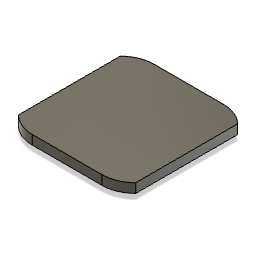
TopPanelWave v5 (Autodesk Fusion 360 design; units mm, degrees)
Autodesk Fusion 360 part; units mm, degrees
sketch "Sketch1" plane through (0, 0, 0) normal (0, 1, 0) x (1, 0, 0)
  line L0 (86, 73.5) -> (-86, 73.5)
  line L1 (-86, 73.5) -> (-86, -73.5)
  line L2 (-86, -73.5) -> (86, -73.5)
  line L3 (86, -73.5) -> (86, 73.5)
  line L4 (86, 73.5) -> (-86, -73.5) construction
  line L5 (-86, 73.5) -> (86, -73.5) construction
  line L6 (-77, -64.5) -> (77, -64.5)
  line L7 (77, -64.5) -> (77, 64.5)
  line L8 (77, 64.5) -> (-77, 64.5)
  line L9 (-77, 64.5) -> (-77, -64.5)
  line L10 (102, -89.5) -> (102, 89.5)
  line L11 (102, 89.5) -> (-102, 89.5)
  line L12 (-102, 89.5) -> (-102, -89.5)
  line L13 (-102, -89.5) -> (102, -89.5)
  dimension "d1" = 172
  dimension "d6" = 147
  dimension "d15" = 16
  constraint horizontal L0
  constraint perpendicular L0 L1
  constraint parallel L0 L2
  constraint parallel L1 L3
  constraint coincident L4 origin
  constraint coincident L5 origin
  measures "d1" distance of L1.end L2.end
  measures "d6" distance of L0.end L1.end
extrude "Extrude1" add sketch "Sketch1" along normal blind 9 contours L0 L1 L2 L3
ref_plane "WorkPlane1" through (0, 9, 0) normal (0, 1, 0) x (0, 0, 1)
sketch "Sketch2" plane through (0, 9, 0) normal (0, 1, 0) x (1, 0, 0)
  line L0 (-77, -64.5) -> (-77, 64.5)
  line L1 (-77, 64.5) -> (77, 64.5)
  line L2 (77, 64.5) -> (77, -64.5)
  line L3 (77, -64.5) -> (-77, -64.5)
  line L4 (86, -73.5) -> (86, 73.5)
  line L5 (86, 73.5) -> (-86, 73.5)
  line L6 (-86, 73.5) -> (-86, -73.5)
  line L7 (-86, -73.5) -> (86, -73.5)
  line L8 (95, -82.5) -> (95, 82.5)
  line L9 (95, 82.5) -> (-95, 82.5)
  line L10 (-95, 82.5) -> (-95, -82.5)
  line L11 (-95, -82.5) -> (95, -82.5)
  line L12 (-111, -98.5) -> (111, -98.5)
  line L13 (111, -98.5) -> (111, 98.5)
  line L14 (111, 98.5) -> (-111, 98.5)
  line L15 (-111, 98.5) -> (-111, -98.5)
  arc A0 (-56.3726, 98.5) -> (-111, 43.8726) centre (-56.3726, 43.8726) ccw
  arc A1 (-111, -43.8726) -> (-56.3726, -98.5) centre (-56.3726, -43.8726) ccw
  arc A2 (56.3726, -98.5) -> (111, -43.8726) centre (56.3726, -43.8726) ccw
  arc A3 (111, 43.8726) -> (56.3726, 98.5) centre (56.3726, 43.8726) ccw
  dimension "d11" = 9
  dimension "d16" = 25
  constraint coincident L9.end A0
  constraint coincident L14 A0.start
  constraint coincident L15 A0.end
  constraint coincident L10.end A1
  constraint coincident L12 A1.end
  constraint coincident L15 A1.start
  constraint coincident L8.start A2
  constraint coincident L13 A2.end
  constraint coincident L12 A2.start
  constraint coincident L8.end A3
  constraint coincident L13 A3.start
  constraint coincident L14 A3.end
  constraint tangent L14 A0
  constraint tangent L15 A0
  constraint tangent L15 A1
  constraint tangent L12 A1
  constraint tangent L12 A2
  constraint tangent L13 A2
  constraint tangent L13 A3
  constraint tangent L14 A3
extrude "Extrude2" add sketch "Sketch2" along normal blind 15 contours L0 L1 L2 L3 | L4 L5 L6 L7 | L8 L9 L10 L11 | L11 L12 A1 A2 | L9 L14 A0 A3
equation "d1 = CaseLength - 2 * SideWidth"
equation "CaseLength = 190 mm"
equation "CaseWidth = 165 mm"
equation "SideWidth = 9 mm"
equation "PanelHeight = 15 mm"
equation "d6 = CaseWidth - 2 * SideWidth"
equation "d7 = -SideWidth"
equation "d8 = SideWidth"
equation "d10 = SideWidth"
equation "d11 = SideWidth"
equation "d12 = PanelHeight"
equation "FlangeWidth = 16 mm"
equation "d15 = FlangeWidth"
equation "d16 = SideWidth + FlangeWidth"
